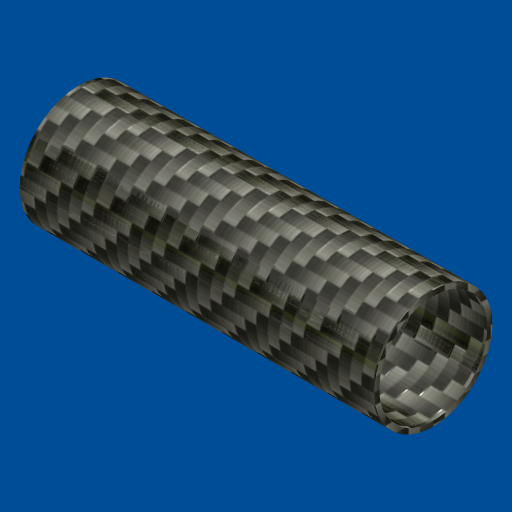
# Autodesk Inventor part: upperArmHinge
Saved by Autodesk Inventor 2023 (Build 270158030, 158C)
## iProperties
Created: 2023-03-03
Part Number: upperArmHinge
Material: CFRP
Document SubType Name: Modeling
Designer: kumpu
Density: 1.43 g/cm^3
Appearance: Carbon Fiber 1
Author: kumpu
Autodesk Inventor part; units mm, degrees
ref_plane "YZ Plane" through (0, 0, 0) normal (1, 0, 0) x (0, 1, 0)
ref_plane "XZ Plane" through (0, 0, 0) normal (0, 1, 0) x (-1, 0, 0)
ref_plane "XY Plane" through (0, 0, 0) normal (0, 0, 1) x (1, 0, 0)
sketch "Sketch1" plane through (0, 0, 0) normal (1, 0, 0) x (0, 1, 0)
  circle A0 centre (0, 0) radius 12.7
  circle A1 centre (0, 0) radius 11.6205
  dimension "d0" = 25.4
  dimension "d1" = 23.241
  constraints: 2 centre point, 2 coincident
  measures "d0" diameter of A0
  measures "d1" diameter of A1
extrude "Extrusion1" add sketch "Sketch1" along normal mid plane 76.2
body "Solid1"
